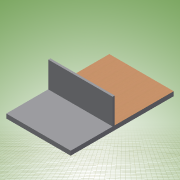
# Autodesk Inventor part: Wall_desk
Saved by Autodesk Inventor 2017 (Build 210142000, 142)
## iProperties
Created: 2018-06-04
Part Number: Wall_desk
Material: Generic
Document SubType Name: Modeling
Designer: Spark Electronics
Density: 1 g/cm^3
Appearance: Default
Author: Spark Electronics
Autodesk Inventor part; units mm, degrees
ref_plane "YZ Plane" through (0, 0, 0) normal (1, 0, 0) x (0, 1, 0)
ref_plane "XZ Plane" through (0, 0, 0) normal (0, 1, 0) x (-1, 0, 0)
ref_plane "XY Plane" through (0, 0, 0) normal (0, 0, 1) x (1, 0, 0)
sketch "Sketch1" plane through (0, 0, 0) normal (0, 0, 1) x (1, 0, 0)
  line L0 (762, -1219.2) -> (-762, -1219.2)
  line L1 (-762, -1219.2) -> (-762, 1219.2)
  line L2 (-762, 1219.2) -> (762, 1219.2)
  line L3 (762, 1219.2) -> (762, -1219.2)
  line L4 (762, -1219.2) -> (-762, 1219.2) construction
  line L5 (-762, -1219.2) -> (762, 1219.2) construction
  point P0 (0, 0)
  dimension "d0" = 1524
  dimension "d5" = 2438.4
  constraints: 12 end point, 2 midpoint, 2 parallel, 1 horizontal, 1 perpendicular
  measures "d0" distance of L1.end L2.end
  measures "d5" distance of L0.end L1.end
extrude "Extrusion1" add sketch "Sketch1" along normal blind 101.6
sketch "Sketch2" plane through (0, 0, 101.6) normal (0, 0, 1) x (1, 0, 0)
  line L0 (-762, -226.9161) -> (762, -226.9161)
  line L1 (762, -226.9161) -> (762, -176.1161)
  line L2 (762, -176.1161) -> (-762, -176.1161)
  line L3 (-762, -176.1161) -> (-762, -226.9161)
  line L4 (-762, 1219.2) -> (-762, -1219.2) projected
  point P0 (0, 0)
  dimension "d6" = 50.8
  dimension "d7" = 1524
  dimension "d8" = 0
  constraints: 8 end point, 2 parallel, 1 horizontal, 1 perpendicular
  measures "d6" distance of L2.end L0.start
  measures "d7" distance of L1.end L2.end
  measures "d8" distance between parallel lines of L4 L3
extrude "Extrusion2" add sketch "Sketch2" along normal blind 609.6
body "Solid1"
